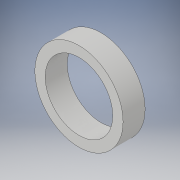
# Autodesk Inventor part: Legs
Saved by Autodesk Inventor 2019 (Build 230136000, 136)
## iProperties
Created: 2021-01-18
Part Number: Legs
Material: Типовые
Document SubType Name: Modeling
Designer: Dazer
Density: 1 g/cm^3
Appearance: По умолчанию
Author: Dazer
## iProperties of the stored document Legs_3DПЕЧАТЬ.ipt
Created: 2021-01-18
Part Number: Legs_3DПЕЧАТЬ
Material: Типовые
Document SubType Name: Modeling
Designer: Dazer
Density: 1 g/cm^3
Appearance: По умолчанию
Author: Dazer
Autodesk Inventor part; units mm, degrees
ref_plane "YZ Plane" through (0, 0, 0) normal (1, 0, 0) x (0, 1, 0)
ref_plane "XZ Plane" through (0, 0, 0) normal (0, 1, 0) x (-1, 0, 0)
ref_plane "XY Plane" through (0, 0, 0) normal (0, 0, 1) x (1, 0, 0)
sketch "Эскиз1" plane through (0, 0, 0) normal (0, 0, 1) x (1, 0, 0)
  circle A0 centre (43.7, 43.7) radius 4.6 projected
  circle A1 centre (43.7, 43.7) radius 6 projected
  circle A2 centre (43.7, -43.7) radius 4.6 projected
  circle A3 centre (43.7, -43.7) radius 6 projected
  circle A4 centre (-43.7, 43.7) radius 4.6 projected
  circle A5 centre (-43.7, 43.7) radius 6 projected
  circle A6 centre (-43.7, -43.7) radius 4.6 projected
  circle A7 centre (-43.7, -43.7) radius 6 projected
  point P0 (0, 0)
extrude "Выдавливание2" add sketch "Эскиз1" along normal blind 2 and the other way blind 1 contours A1
